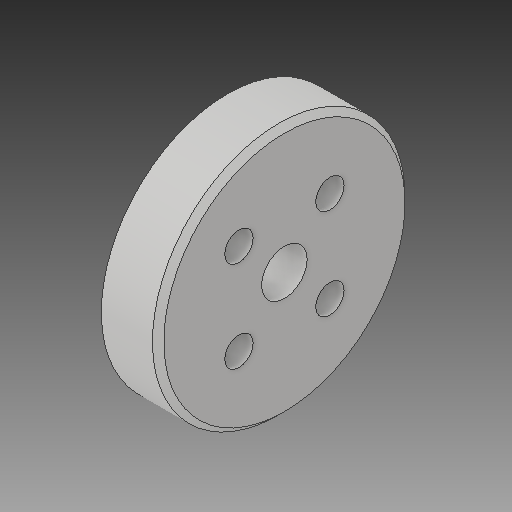
# Autodesk Inventor part: Tapon 2
Saved by Autodesk Inventor 2018.3 (Build 223284000, 284)
## iProperties
Created: 2019-03-13
Part Number: Tapon 2
Material: Generic
Document SubType Name: Modeling
Designer: Mario
Density: 1 g/cm^3
Appearance: Default
Author: Mario
Autodesk Inventor part; units mm, degrees
ref_plane "YZ Plane" through (0, 0, 0) normal (1, 0, 0) x (0, 1, 0)
ref_plane "XZ Plane" through (0, 0, 0) normal (0, 1, 0) x (-1, 0, 0)
ref_plane "XY Plane" through (0, 0, 0) normal (0, 0, 1) x (1, 0, 0)
sketch "Sketch1" plane through (0, 0, 0) normal (1, 0, 0) x (0, 1, 0)
  circle A0 centre (0, 0) radius 22.2155
  circle A1 centre (0, 0) radius 22.2155 projected
  dimension "d20" = 44.431
  dimension "d21" = 44.431
  constraints: 1 centre point, 1 coincident
  measures "d20" diameter of A1
  measures "d21" diameter of A0
extrude "Extrusion1" add sketch "Sketch1" along normal blind 10
sketch "Sketch2" plane through (0, 0, 0) normal (-1, 0, 0) x (0, 0, 1)
  point P0 (0, 0)
  point P1 (8, 8)
  point P2 (8, -8)
  point P3 (-8, -8)
  point P4 (-8, 8)
  dimension "d2" = 8
  dimension "d3" = 8
  dimension "d4" = 16
  dimension "d5" = 16
  constraints: 2 horizontal alignment, 2 vertical alignment
  measures "d2" horizontal distance of point (8, 8) point (0, 0)
  measures "d3" horizontal distance of point (0, 0) point (8, 8)
  measures "d4" distance of point (8, 8) point (-8, 8)
  measures "d5" distance of point (-8, -8) point (-8, 8)
hole "Hole1" at (0, 8, 8) at (0, -8, 8) at (0, -8, -8) at (0, 8, -8) direction (1, 0, 0) diameter 5 end through all
sketch "Sketch3" plane through (0, 0, 0) normal (-1, 0, 0) x (0, 0, 1)
  point P0 (0, 0)
  point P1 (0, 0)
  constraints: 1 coincident
hole "Hole2" at (0, 0, 0) direction (1, 0, 0) diameter 8 end through all
chamfer "Chamfer2" distance 1 distance2 1 1 edges at (10, -22.2155, 0) measured on face at (10, -21.7155, 0)
equation "\"d21\" = d20"
equation "\"d4\" = 2 * d2"
equation "\"d5\" = d4"
body "Solid1"
